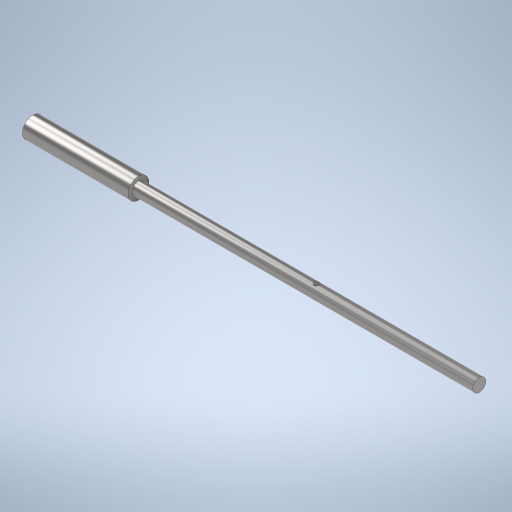
# Autodesk Inventor part: wormgear_axis_6mm
Saved by Autodesk Inventor 2024 (Build 280153000, 153)
## iProperties
Created: 2025-12-09
Part Number: wormgear_axis_6mm
Material: Stainless Steel
Document SubType Name: Modeling
Designer: schar
Density: 8 g/cm^3
Appearance: Semi-Polished
Author: schar
Autodesk Inventor part; units mm, degrees
ref_plane "YZ Plane" through (0, 0, 0) normal (1, 0, 0) x (0, 1, 0)
ref_plane "XZ Plane" through (0, 0, 0) normal (0, 1, 0) x (-1, 0, 0)
ref_plane "XY Plane" through (0, 0, 0) normal (0, 0, 1) x (1, 0, 0)
sketch "Sketch1" plane through (0, 0, 0) normal (1, 0, 0) x (0, 1, 0)
  circle A0 centre (0, 0) radius 4
  circle A1 centre (0, 0) radius 2.5
  line L0 (2, 0) -> (2, -1.5)
  line L1 (2, 0) -> (2, 1.5)
  dimension "d0" = 8
  dimension "d1" = 5
  constraints: 4 end point, 2 centre point, 2 coincident, 2 point on circle, 1 point on line
  measures "d0" diameter of A0
  measures "d1" diameter of A1
extrude "Extrusion1" add sketch "Sketch1" along normal blind 8 contours A0 | A1 L0 L1 picked at (2.0912, -0.8466)
sketch "Sketch2" plane through (8, 0, 0) normal (1, 0, 0) x (0, 0, -1)
  circle A0 centre (0, 0) radius 4
  circle A1 centre (0, 0) radius 2.5
  constraints: 2 centre point, 2 coincident
extrude "Extrusion2" add sketch "Sketch2" along normal blind 2
sketch "Sketch3" plane through (8, 0, 0) normal (1, 0, 0) x (0, 0, -1)
  circle A0 centre (0, 0) radius 2.5
  constraints: 1 centre point, 1 coincident
extrude "Extrusion3" add sketch "Sketch3" along normal blind 151
sketch "Sketch4" plane through (0, 0, 0) normal (-1, 0, 0) x (0, 0, 1)
  circle A0 centre (0, 0) radius 4
  constraints: 1 centre point, 1 coincident
extrude "Extrusion4" cut sketch "Sketch4" against normal blind 2.5
sketch "Sketch6" plane through (0, 0, 0) normal (0, 1, 0) x (-1, 0, 0)
  line L0 (-159, 2.5) -> (-159, -2.5) projected
  line L1 (-159, 0) -> (-96, 0)
  circle A0 centre (-96, 0) radius 1
  point P0 (0, 0)
  dimension "d17" = 63
  dimension "d18" = 2
  constraints: 2 end point, 1 centre point, 1 coincident, 1 horizontal, 1 midpoint
  measures "d17" distance of L1.start L1.end
  measures "d18" diameter of A0
extrude "Extrusion6" cut sketch "Sketch6" along normal blind 10
thread "Thread2" size "M2x0.4" class "6H" standard "ANSI Metric M Profile" full length
sketch "Sketch7" plane through (2.5, 0, 0) normal (-1, 0, 0) x (0, 0, 1)
  circle A0 centre (0, 0) radius 2.5
  circle A1 centre (0, 0) radius 4
  line L0 (1.5, 2) -> (-1.5, 2) projected
  line L1 (0, 2) -> (1.5, 2)
  line L2 (0, 2) -> (-1.5, 2)
  constraints: 4 end point, 2 centre point, 2 coincident, 2 collinear, 1 midpoint
extrude "Extrusion7" add sketch "Sketch7" along normal blind 16.5
sketch "Sketch8" plane through (2.5, 0, 0) normal (-1, 0, 0) x (0, 0, 1)
  circle A0 centre (0, 0) radius 2.5
  line L0 (1.5, 2) -> (-1.5, 2) projected
  line L1 (1.5, 2) -> (-1.5, 2)
  constraints: 2 end point, 1 centre point, 1 coincident, 1 horizontal
extrude "Extrusion8" add sketch "Sketch8" along normal blind 16.5 contours L0 A0 picked at (-0.3466, 2.0912)
sketch "Sketch10" plane through (10, 0, 0) normal (1, 0, 0) x (0, 0, -1)
  circle A0 centre (0, 0) radius 2.5
  circle A1 centre (0, 0) radius 4
  constraints: 2 centre point, 2 coincident
extrude "Extrusion9" add sketch "Sketch10" along normal blind 17
body "Solid1"
